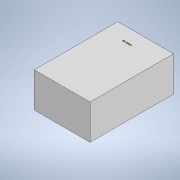
# Autodesk Inventor part: PX9200-23A_LIPO_Battery
Saved by Autodesk Inventor 2022.3 (Build 263350000, 350)
## iProperties
Created: 2022-07-07
Part Number: PX9200-23A_LIPO_Battery
Material: Generic
Document SubType Name: Modeling
Designer: luis_
Density: 1 g/cm^3
Appearance: Default
Author: luis_
Autodesk Inventor part; units mm, degrees
ref_plane "YZ Plane" through (0, 0, 0) normal (1, 0, 0) x (0, 1, 0)
ref_plane "XZ Plane" through (0, 0, 0) normal (0, 1, 0) x (-1, 0, 0)
ref_plane "XY Plane" through (0, 0, 0) normal (0, 0, 1) x (1, 0, 0)
extrude "Extrusion1" [suppressed]
sketch "Sketch2" plane through (-76.454, 0, 51.054) normal (0, 0, 1) x (1, 0, 0)
  point P0 (76.454, 0)
sketch "Sketch3" plane through (0, 0, 0) normal (0, 0, 1) x (1, 0, 0)
  line L0 (-51.054, -32.004) -> (51.054, -32.004)
  line L1 (51.054, -32.004) -> (51.054, 32.004)
  line L2 (51.054, 32.004) -> (-51.054, 32.004)
  line L3 (-51.054, 32.004) -> (-51.054, -32.004)
  line L4 (-51.054, -32.004) -> (51.054, 32.004) construction
  line L5 (51.054, -32.004) -> (-51.054, 32.004) construction
  point P0 (0, 0)
  dimension "d4" = 102.108
  dimension "d5" = 64.008
  constraints: 12 end point, 2 midpoint, 2 parallel, 1 horizontal, 1 perpendicular
  measures "d4" distance of L2.end L1.end
  measures "d5" distance of L1.end L0.end
extrude "Extrusion2" add sketch "Sketch3" against normal blind 152.908
sketch "Sketch4" plane through (-51.054, 32.004, 0) normal (0, 1, 0) x (1, 0, 0)
  line L0 (34.4174, 129.0093) -> (73.7734, 129.0093) construction
  line L1 (73.7734, 129.0093) -> (73.7734, 25.3554) construction
  line L2 (73.7734, 25.3554) -> (34.4174, 25.3554) construction
  line L3 (34.4174, 25.3554) -> (34.4174, 129.0093) construction
  point P0 (51.054, 0)
  constraints: 2 other
body "Solid1"
